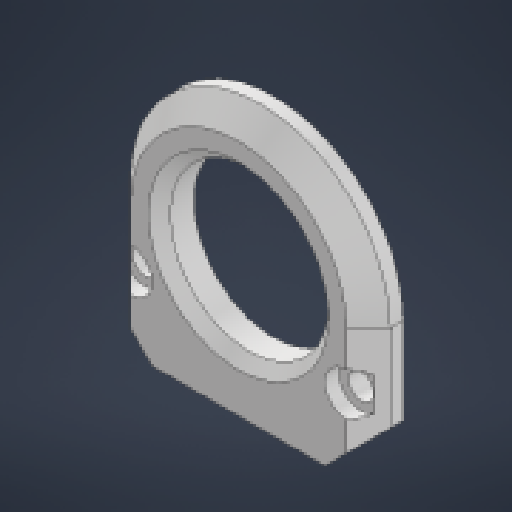
# Autodesk Inventor part: Venstre_bearing_lock
Saved by Autodesk Inventor 2023.4 (Build 274418000, 418)
## iProperties
Created: 2025-09-28
Part Number: Venstre_bearing_lock
Material: Generic
Document SubType Name: Modeling
Designer: Malthe Sennels
Density: 1 g/cm^3
Appearance: Default
Author: Malthe Sennels
Autodesk Inventor part; units mm, degrees
ref_plane "YZ Plane" through (0, 0, 0) normal (1, 0, 0) x (0, 1, 0)
ref_plane "XZ Plane" through (0, 0, 0) normal (0, 1, 0) x (-1, 0, 0)
ref_plane "XY Plane" through (0, 0, 0) normal (0, 0, 1) x (1, 0, 0)
sketch "Sketch1" plane through (0, 0, 0) normal (0, 0, 1) x (1, 0, 0)
  circle A0 centre (0, 0) radius 13.125 projected
  line L0 (18, -12) -> (12, -18) projected
  line L1 (18, 0) -> (18, -12) projected
  arc A1 (18, 0) -> (-18, 0) centre (0, 0) ccw projected
  line L2 (-18, -12) -> (-18, 0) projected
  line L3 (-12, -18) -> (-18, -12) projected
  line L4 (12, -18) -> (-12, -18) projected
  line L5 (-15, -69.1421) -> (15, -69.1421) projected
  circle A2 centre (0, 0) radius 12.5 projected
  circle A3 centre (0, 0) radius 11
  circle A4 centre (15, -7.9289) radius 1.75 projected
  circle A5 centre (-15, -7.9289) radius 1.75 projected
  line L6 (-15, -10.1789) -> (-15, -69.1421) projected
  line L7 (-15, -10.1789) -> (-12.75, -10.1789) projected
  line L8 (-12.75, -10.1789) -> (-12.75, -5.6789) projected
  line L9 (-12.75, -5.6789) -> (-15, -5.6789) projected
  line L10 (-15, 0) -> (-15, -5.6789) projected
  arc A6 (15, 0) -> (-15, 0) centre (0, 0) ccw projected
  line L11 (15, -5.6789) -> (15, 0) projected
  line L12 (15, -5.6789) -> (12.75, -5.6789) projected
  line L13 (12.75, -5.6789) -> (12.75, -10.1789) projected
  line L14 (12.75, -10.1789) -> (15, -10.1789) projected
  line L15 (15, -69.1421) -> (15, -10.1789) projected
  point P0 (0, 0)
  constraints: 1 centre point, 2 other
ref_plane "Work Plane1" through (-15, -65, 4.85) normal (0, 0, 1) x (1, 0, 0)
extrude "Extrusion1" add sketch "Sketch1" along normal up to surface (4.85 mm away) contours A0 | L0 L15 L14 L13 L12 L11 A6 L10 L9 L8 L7 L6 L3 L2 A1 L1 | L0 L4 L3 L6 L7 L8 L9 L10 A6 L11 L12 L13 L14 L15 | A2 | A4 | A5
chamfer "Chamfer1" distance 3 angle 45 3 edges at (-18, -6, 4.85) (0, 18, 4.85) (18, -6, 4.85)
chamfer "Chamfer2" distance 1.5 angle 45 1 edges at (-11, 0, 4.85)
sketch "Sketch2" plane through (-12, -18, 4.85) normal (0, 0, 1) x (1, 0, 0)
  circle A0 centre (27, 10.0711) radius 1.75 projected
  circle A1 centre (-3, 10.0711) radius 1.75 projected
  point P0 (12, 18)
extrude "Extrusion2" cut sketch "Sketch2" against normal through all
sketch "Sketch3" plane through (-12, -18, 4.85) normal (0, 0, 1) x (1, 0, 0)
  circle A0 centre (-3, 10.0711) radius 1.75 projected
  circle A1 centre (-3, 10.0711) radius 3
  arc A2 (27, 11.8211) -> (27, 8.3211) centre (27, 10.0711) ccw projected
  circle A3 centre (27, 10.0711) radius 3
  point P0 (12, 18)
  dimension "d10" = 6
  dimension "d11" = 6
  constraints: 2 centre point, 2 coincident
  measures "d10" diameter of A1
  measures "d11" diameter of A3
extrude "Extrusion3" cut sketch "Sketch3" against normal blind 2 contours A0 | A1 | A3
body "Solid1"
